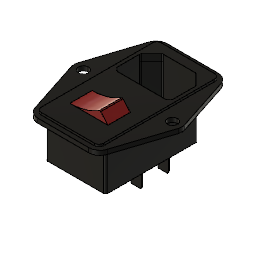
RM PSU Assembly (Autodesk Fusion 360 archive; units mm, degrees)
design "IEC Inlet"
Autodesk Fusion 360 part; units mm, degrees
(part 1 of 2)
sketch "Sketch1" plane through (0, 0, 0) normal (0, 0, 1) x (1, 0, 0)
  line L0 (-25, 14) -> (25, 14)
  line L1 (27, 12) -> (27, -12)
  line L2 (25, -14) -> (-25, -14)
  line L3 (-27, -12) -> (-27, 12)
  arc A0 (-25, 14) -> (-27, 12) centre (-25, 12) ccw
  arc A1 (-27, -12) -> (-25, -14) centre (-25, -12) ccw
  arc A2 (25, -14) -> (27, -12) centre (25, -12) ccw
  arc A3 (27, 12) -> (25, 14) centre (25, 12) ccw
  dimension "d1" = 28
  dimension "d2" = 54
  dimension "d3" = 14
  dimension "d4" = 27
  dimension "d5" = 2
  constraint horizontal L0
  constraint vertical L1
  constraint horizontal L2
  constraint vertical L3
  constraint tangent L3 A0
  constraint tangent L0 A0
  constraint tangent L3 A1
  constraint tangent L2 A1
  constraint equal A0 A1
  constraint tangent L2 A2
  constraint tangent L1 A2
  constraint equal A0 A2
  constraint tangent L1 A3
  constraint tangent L0 A3
  constraint equal A0 A3
  measures "d1" distance of L0 L2
  measures "d2" distance of L1 L3
  measures "d3" distance of origin L2
  measures "d4" distance of origin L3
  measures "d5" radius of A0
extrude "Extrude1" add sketch "Sketch1" along normal blind 1
sketch "Sketch2" plane through (0, 0, 0) normal (0, 0, -1) x (1, 0, 0)
  arc A0 (27, 12) -> (25, 14) centre (25, 12) ccw
  line L0 (25, 14) -> (-25, 14)
  arc A1 (-25, 14) -> (-27, 12) centre (-25, 12) ccw
  line L1 (-27, 12) -> (-27, -12)
  arc A2 (-27, -12) -> (-25, -14) centre (-25, -12) ccw
  line L2 (-25, -14) -> (25, -14)
  arc A3 (25, -14) -> (27, -12) centre (25, -12) ccw
  line L3 (27, -12) -> (27, 12)
  line L4 (-29, 24.5) -> (29, 24.5)
  line L5 (29, 11.423) -> (29, -11.423)
  line L6 (29, -24.5) -> (-29, -24.5)
  line L7 (-29, -11.423) -> (-29, 11.423)
  circle A4 centre (0, -20) radius 2.25
  circle A5 centre (0, 20) radius 2.25
  line L8 (1.5487, -23.9955) -> (25.5487, -16.1771)
  line L9 (-1.5487, -23.9955) -> (-25.5487, -16.1771)
  line L10 (1.5487, 23.9955) -> (25.5487, 16.1771)
  line L11 (-1.5487, 23.9955) -> (-25.5487, 16.1771)
  arc A6 (25.5487, -16.1771) -> (29, -11.423) centre (24, -11.423) ccw
  arc A7 (29, 11.423) -> (25.5487, 16.1771) centre (24, 11.423) ccw
  arc A8 (-25.5487, 16.1771) -> (-29, 11.423) centre (-24, 11.423) ccw
  arc A9 (-29, -11.423) -> (-25.5487, -16.1771) centre (-24, -11.423) ccw
  arc A10 (-1.5487, -23.9955) -> (1.5487, -23.9955) centre (0, -19.2414) ccw
  arc A11 (1.5487, 23.9955) -> (-1.5487, 23.9955) centre (0, 19.2414) ccw
  point P0 (0, -24.5)
  point P1 (29, -15.0528)
  point P2 (-29, -15.0528)
  point P3 (0, 24.5)
  point P4 (29, 15.0528)
  point P5 (-29, 15.0528)
  dimension "d8" = 58
  dimension "d9" = 29
  dimension "d10" = 49
  dimension "d11" = 24.5
  dimension "d12" = 4.5
  dimension "d13" = 4.5
  dimension "d14" = 40
  dimension "d15" = 4.5
  dimension "d16" = 30.5
  dimension "d17" = 30.5
  dimension "d18" = 30.5
  dimension "d19" = 30.5
  dimension "d20" = 5
  dimension "d21" = 5
  constraint horizontal L4
  constraint vertical L5
  constraint horizontal L6
  constraint vertical L7
  constraint vertical origin A5.centre
  constraint vertical origin A4.centre
  constraint midpoint L6 P0
  constraint coincident L5 P1
  constraint coincident L7 P2
  constraint midpoint L4 P3
  constraint coincident L5 P4
  constraint coincident L7 P5
  constraint coincident P1 L8
  constraint coincident L6.start L5
  constraint tangent L8 A6
  constraint tangent L5 A6
  constraint coincident L4.end L5
  constraint coincident P4 L10
  constraint tangent L5 A7
  constraint tangent L10 A7
  constraint equal A6 A7
  constraint coincident P5 L11
  constraint coincident L4.start L7
  constraint tangent L11 A8
  constraint tangent L7 A8
  constraint equal A6 A8
  constraint coincident L6.end L7
  constraint coincident P2 L9
  constraint tangent L7 A9
  constraint tangent L9 A9
  constraint equal A6 A9
  constraint coincident P0 L9
  constraint coincident P0 L8
  constraint tangent L9 A10
  constraint tangent L8 A10
  constraint coincident P3 L10
  constraint coincident P3 L11
  constraint tangent L10 A11
  constraint tangent L11 A11
  constraint equal A10 A11
  measures "d8" distance of L5 L7
  measures "d9" distance of origin L7
  measures "d10" distance of L4 L6
  measures "d11" distance of origin L6
  measures "d12" diameter of A4
  measures "d13" diameter of A5
  measures "d14" distance of A4.centre A5.centre
  measures "d15" distance of L6 A4.centre
  measures "d16" distance of P0 P1
  measures "d17" distance of P0 P2
  measures "d18" distance of P3 P4
  measures "d19" distance of P3 P5
  measures "d20" radius of A6
  measures "d21" radius of A10
extrude "Extrude2" add sketch "Sketch2" along normal blind 2 contours A0 L0 A1 L1 A2 L2 A3 L3 | L5 L7 L8 L9 L10 L11 A6 A7 A8 A9 A10 A11
sketch "Sketch3" plane through (0, 0, -2) normal (0, 0, -1) x (1, 0, 0)
  circle A0 centre (0, 20) radius 2.25
  circle A1 centre (0, -20) radius 2.25
  arc A2 (29, 11.423) -> (25.5487, 16.1771) centre (24, 11.423) ccw
  line L0 (25.5487, 16.1771) -> (1.5487, 23.9955)
  arc A3 (1.5487, 23.9955) -> (-1.5487, 23.9955) centre (0, 19.2414) ccw
  line L1 (-1.5487, 23.9955) -> (-25.5487, 16.1771)
  arc A4 (-25.5487, 16.1771) -> (-29, 11.423) centre (-24, 11.423) ccw
  line L2 (-29, 11.423) -> (-29, -11.423)
  arc A5 (-29, -11.423) -> (-25.5487, -16.1771) centre (-24, -11.423) ccw
  line L3 (-25.5487, -16.1771) -> (-1.5487, -23.9955)
  arc A6 (-1.5487, -23.9955) -> (1.5487, -23.9955) centre (0, -19.2414) ccw
  line L4 (1.5487, -23.9955) -> (25.5487, -16.1771)
  arc A7 (25.5487, -16.1771) -> (29, -11.423) centre (24, -11.423) ccw
  line L5 (29, -11.423) -> (29, 11.423)
  line L6 (-22.5, 13.5) -> (22.5, 13.5)
  line L7 (23.5, 12.5) -> (23.5, -12.5)
  line L8 (22.5, -13.5) -> (-22.5, -13.5)
  line L9 (-23.5, -12.5) -> (-23.5, 12.5)
  arc A8 (23.5, 12.5) -> (22.5, 13.5) centre (22.5, 12.5) ccw
  arc A9 (22.5, -13.5) -> (23.5, -12.5) centre (22.5, -12.5) ccw
  arc A10 (-23.5, -12.5) -> (-22.5, -13.5) centre (-22.5, -12.5) ccw
  arc A11 (-22.5, 13.5) -> (-23.5, 12.5) centre (-22.5, 12.5) ccw
  dimension "d24" = 27
  dimension "d25" = 47
  dimension "d26" = 23.5
  dimension "d27" = 13.5
  dimension "d30" = 1
  constraint horizontal L6
  constraint vertical L7
  constraint horizontal L8
  constraint vertical L9
  constraint tangent L6 A8
  constraint tangent L7 A8
  constraint tangent L7 A9
  constraint tangent L8 A9
  constraint equal A8 A9
  constraint tangent L8 A10
  constraint tangent L9 A10
  constraint equal A8 A10
  constraint tangent L9 A11
  constraint tangent L6 A11
  constraint equal A8 A11
  measures "d24" distance of L6 L8
  measures "d25" distance of L7 L9
  measures "d26" distance of origin L9
  measures "d27" distance of origin L6
  measures "d30" radius of A8
extrude "Extrude3" add sketch "Sketch3" along normal blind 18 contours L6 L7 L8 L9 A8 A9 A10 A11
sketch "Sketch4" plane through (0, 0, -20) normal (0, 0, -1) x (1, 0, 0)
  arc A0 (23.5, 12.5) -> (22.5, 13.5) centre (22.5, 12.5) ccw
  line L0 (22.5, 13.5) -> (-22.5, 13.5)
  arc A1 (-22.5, 13.5) -> (-23.5, 12.5) centre (-22.5, 12.5) ccw
  line L1 (-23.5, 12.5) -> (-23.5, -12.5)
  arc A2 (-23.5, -12.5) -> (-22.5, -13.5) centre (-22.5, -12.5) ccw
  line L2 (-22.5, -13.5) -> (22.5, -13.5)
  arc A3 (22.5, -13.5) -> (23.5, -12.5) centre (22.5, -12.5) ccw
  line L3 (23.5, -12.5) -> (23.5, 12.5)
  line L4 (17.136, 13.5) -> (23.5, 7.136)
  line L5 (23.5, -7.136) -> (17.136, -13.5)
  dimension "d31" = 9
  dimension "d32" = 9
  dimension "d33" = 45
  dimension "d34" = 45
  constraint coincident L0 L4.start
  constraint coincident L3 L4.end
  constraint coincident L3 L5.start
  constraint coincident L2 L5.end
  measures "d31" distance of L5.start L5.end
  measures "d32" distance of L4.start L4.end
  measures "d33" angle of L3 L4
  measures "d34" angle of L3 L5
extrude "Extrude4" cut sketch "Sketch4" against normal blind 18 contours A0 L0 L3 L4 | L2 A3 L3 L5
sketch "Sketch5" plane through (0, 0, 1) normal (0, 0, 1) x (-1, 0, 0)
  arc A0 (-25, 14) -> (-27, 12) centre (-25, 12) ccw
  line L0 (-27, 12) -> (-27, -12)
  arc A1 (-27, -12) -> (-25, -14) centre (-25, -12) ccw
  line L1 (-25, -14) -> (25, -14)
  arc A2 (25, -14) -> (27, -12) centre (25, -12) ccw
  line L2 (27, -12) -> (27, 12)
  arc A3 (27, 12) -> (25, 14) centre (25, 12) ccw
  line L3 (25, 14) -> (-25, 14)
  line L4 (-8, -12.5) -> (-17.636, -12.5)
  line L5 (-23, -7.136) -> (-23, 7.136)
  line L6 (-17.636, 12.5) -> (-8, 12.5)
  line L7 (-6, 10.5) -> (-6, -10.5)
  line L8 (-18.3431, 12.2071) -> (-22.7071, 7.8431)
  line L9 (-22.7071, -7.8431) -> (-18.3431, -12.2071)
  arc A4 (-8, -12.5) -> (-6, -10.5) centre (-8, -10.5) ccw
  arc A5 (-6, 10.5) -> (-8, 12.5) centre (-8, 10.5) ccw
  arc A6 (-18.3431, -12.2071) -> (-17.636, -12.5) centre (-17.636, -11.5) ccw
  arc A7 (-23, -7.136) -> (-22.7071, -7.8431) centre (-22, -7.136) ccw
  arc A8 (-22.7071, 7.8431) -> (-23, 7.136) centre (-22, 7.136) ccw
  arc A9 (-17.636, 12.5) -> (-18.3431, 12.2071) centre (-17.636, 11.5) ccw
  point P0 (-18.0503, 12.5)
  point P1 (-23, 7.5503)
  point P2 (-23, -7.5503)
  point P3 (-18.0503, -12.5)
  dimension "d37" = 4
  dimension "d38" = 17
  dimension "d39" = 25
  dimension "d40" = 12.5
  dimension "d41" = 7
  dimension "d42" = 7
  dimension "d43" = 45
  dimension "d44" = 45
  dimension "d45" = 2
  dimension "d46" = 1
  constraint horizontal L4
  constraint vertical L5
  constraint horizontal L6
  constraint vertical L7
  constraint coincident L6 P0
  constraint coincident L5 P1
  constraint coincident L5 P2
  constraint coincident L4 P3
  constraint tangent L4 A4
  constraint tangent L7 A4
  constraint tangent L6 A5
  constraint tangent L7 A5
  constraint equal A4 A5
  constraint coincident P3 L9
  constraint tangent L4 A6
  constraint tangent L9 A6
  constraint coincident P2 L9
  constraint tangent L9 A7
  constraint tangent L5 A7
  constraint equal A6 A7
  constraint coincident P1 L8
  constraint tangent L5 A8
  constraint tangent L8 A8
  constraint equal A6 A8
  constraint coincident P0 L8
  constraint tangent L8 A9
  constraint tangent L6 A9
  constraint equal A6 A9
  measures "d37" distance of L0 L5
  measures "d38" distance of L5 L7
  measures "d39" distance of L4 L6
  measures "d40" distance of origin L6
  measures "d41" distance of P0 P1
  measures "d42" distance of P2 P3
  measures "d43" angle of L5 L9
  measures "d44" angle of L5 L8
  measures "d45" radius of A4
  measures "d46" radius of A6
extrude "Extrude5" cut sketch "Sketch5" against normal blind 18 contours L4 L5 L6 L7 L8 L9 A4 A5 A6 A7 A8 A9
sketch "Sketch6" plane through (0, 0, 1) normal (0, 0, 1) x (-1, 0, 0)
  line L0 (-17.636, 12.5) -> (-8, 12.5)
  arc A0 (-6, 10.5) -> (-8, 12.5) centre (-8, 10.5) ccw
  line L1 (-6, 10.5) -> (-6, -10.5)
  arc A1 (-8, -12.5) -> (-6, -10.5) centre (-8, -10.5) ccw
  line L2 (-8, -12.5) -> (-17.636, -12.5)
  arc A2 (-18.3431, -12.2071) -> (-17.636, -12.5) centre (-17.636, -11.5) ccw
  line L3 (-18.3431, -12.2071) -> (-22.7071, -7.8431)
  arc A3 (-23, -7.136) -> (-22.7071, -7.8431) centre (-22, -7.136) ccw
  line L4 (-23, -7.136) -> (-23, 7.136)
  arc A4 (-22.7071, 7.8431) -> (-23, 7.136) centre (-22, 7.136) ccw
  line L5 (-22.7071, 7.8431) -> (-18.3431, 12.2071)
  arc A5 (-17.636, 12.5) -> (-18.3431, 12.2071) centre (-17.636, 11.5) ccw
  arc A6 (-25, 14) -> (-27, 12) centre (-25, 12) ccw
  line L6 (-27, 12) -> (-27, -12)
  arc A7 (-27, -12) -> (-25, -14) centre (-25, -12) ccw
  line L7 (-25, -14) -> (25, -14)
  arc A8 (25, -14) -> (27, -12) centre (25, -12) ccw
  line L8 (27, -12) -> (27, 12)
  arc A9 (27, 12) -> (25, 14) centre (25, 12) ccw
  line L9 (25, 14) -> (-25, 14)
  line L10 (17, -8) -> (7, -8)
  line L11 (7, -8) -> (7, 8)
  line L12 (7, 8) -> (17, 8)
  line L13 (17, 8) -> (17, -8)
  line L14 (17, 4.5) -> (7, 4.5)
  dimension "d49" = 16
  dimension "d50" = 10
  dimension "d51" = 10
  dimension "d52" = 6
  dimension "d53" = 12.5
  constraint horizontal L10
  constraint vertical L11
  constraint horizontal L12
  constraint vertical L13
  constraint coincident L13 L14.start
  constraint coincident L11 L14.end
  constraint perpendicular L11 L14
  measures "d49" distance of L10 L12
  measures "d50" distance of L11 L13
  measures "d51" distance of L8 L13
  measures "d52" distance of L7 L10
  measures "d53" distance of L10 L14
extrude "Extrude6" add sketch "Sketch6" along normal blind 4 contours L11 L12 L13 L14
fillet "Fillet1" radius 25 1 edges at (-12, -4.5, 1)
sketch "Sketch7" plane through (-17, 0, 0) normal (-1, 0, 0) x (0, -1, 0)
  line L0 (-9.0647, 1) -> (8, 1)
  line L1 (8, 1) -> (8, 5)
  line L2 (8, 5) -> (4.5, 5)
  arc A0 (-9.0647, 1) -> (4.5, 5) centre (-9.0647, 26) ccw
  line L3 (4.5, 5) -> (8, 1)
  constraint coincident L2.end A0.end
  constraint coincident L0.end L1.start
extrude "Extrude7" cut sketch "Sketch7" against normal blind 10 contours L1 L2 L3
fillet "Fillet2" radius 0.5 1 edges at (-12, -4.5, 5)
sketch "Sketch9" plane through (0, 0, -20) normal (0, 0, -1) x (1, 0, 0)
  line L0 (23.5, 7.136) -> (17.136, 13.5)
  line L1 (17.136, 13.5) -> (-22.5, 13.5)
  arc A0 (-22.5, 13.5) -> (-23.5, 12.5) centre (-22.5, 12.5) ccw
  line L2 (-23.5, 12.5) -> (-23.5, -12.5)
  arc A1 (-23.5, -12.5) -> (-22.5, -13.5) centre (-22.5, -12.5) ccw
  line L3 (-22.5, -13.5) -> (17.136, -13.5)
  line L4 (17.136, -13.5) -> (23.5, -7.136)
  line L5 (23.5, -7.136) -> (23.5, 7.136)
  line L6 (-21.5, 12.5) -> (-8.5, 12.5)
  line L7 (-7.5, 11.5) -> (-7.5, -11.5)
  line L8 (-8.5, -12.5) -> (-21.5, -12.5)
  line L9 (-22.5, -11.5) -> (-22.5, 11.5)
  arc A2 (-21.5, 12.5) -> (-22.5, 11.5) centre (-21.5, 11.5) ccw
  arc A3 (-7.5, 11.5) -> (-8.5, 12.5) centre (-8.5, 11.5) ccw
  arc A4 (-8.5, -12.5) -> (-7.5, -11.5) centre (-8.5, -11.5) ccw
  arc A5 (-22.5, -11.5) -> (-21.5, -12.5) centre (-21.5, -11.5) ccw
  dimension "d62" = 1
  dimension "d63" = 1
  dimension "d64" = 1
  dimension "d65" = 15
  dimension "d66" = 1
  constraint horizontal L6
  constraint vertical L7
  constraint horizontal L8
  constraint vertical L9
  constraint tangent L6 A2
  constraint tangent L9 A2
  constraint tangent L6 A3
  constraint tangent L7 A3
  constraint equal A2 A3
  constraint tangent L7 A4
  constraint tangent L8 A4
  constraint equal A2 A4
  constraint tangent L8 A5
  constraint tangent L9 A5
  constraint equal A2 A5
  measures "d62" distance of L1 L6
  measures "d63" distance of L3 L8
  measures "d64" distance of L2 L9
  measures "d65" distance of L7 L9
  measures "d66" radius of A2
extrude "Extrude8" cut sketch "Sketch9" against normal blind 18 contours L6 L7 L8 L9 A2 A3 A4 A5
sketch "Sketch10" plane through (0, 0, -20) normal (0, 0, -1) x (1, 0, 0)
  line L0 (-22.5, -11.5) -> (-22.5, 11.5)
  arc A0 (-21.5, 12.5) -> (-22.5, 11.5) centre (-21.5, 11.5) ccw
  line L1 (-21.5, 12.5) -> (-8.5, 12.5)
  arc A1 (-7.5, 11.5) -> (-8.5, 12.5) centre (-8.5, 11.5) ccw
  line L2 (-7.5, 11.5) -> (-7.5, -11.5)
  arc A2 (-8.5, -12.5) -> (-7.5, -11.5) centre (-8.5, -11.5) ccw
  line L3 (-8.5, -12.5) -> (-21.5, -12.5)
  arc A3 (-22.5, -11.5) -> (-21.5, -12.5) centre (-21.5, -11.5) ccw
  line L4 (23.5, 7.136) -> (17.136, 13.5)
  line L5 (17.136, 13.5) -> (-22.5, 13.5)
  arc A4 (-22.5, 13.5) -> (-23.5, 12.5) centre (-22.5, 12.5) ccw
  line L6 (-23.5, 12.5) -> (-23.5, -12.5)
  arc A5 (-23.5, -12.5) -> (-22.5, -13.5) centre (-22.5, -12.5) ccw
  line L7 (-22.5, -13.5) -> (17.136, -13.5)
  line L8 (17.136, -13.5) -> (23.5, -7.136)
  line L9 (23.5, -7.136) -> (23.5, 7.136)
  line L10 (19.5, 2.5) -> (20, 2.5)
  line L11 (20, 2.5) -> (20, -2.5)
  line L12 (20, -2.5) -> (19.5, -2.5)
  line L13 (19.5, -2.5) -> (19.5, 2.5)
  line L14 (8.636, 9.5) -> (9.136, 9.5)
  line L15 (9.136, 9.5) -> (9.136, 4.5)
  line L16 (9.136, 4.5) -> (8.636, 4.5)
  line L17 (8.636, 4.5) -> (8.636, 9.5)
  line L18 (-3.364, 9.5) -> (-2.864, 9.5)
  line L19 (-2.864, 9.5) -> (-2.864, 4.5)
  line L20 (-2.864, 4.5) -> (-3.364, 4.5)
  line L21 (-3.364, 4.5) -> (-3.364, 9.5)
  dimension "d69" = 5
  dimension "d70" = 0.5
  dimension "d71" = 0.5
  dimension "d72" = 5
  dimension "d75" = 3.5
  dimension "d76" = 11
  dimension "d77" = 4
  dimension "d78" = 5
  dimension "d79" = 0.5
  dimension "d80" = 4
  dimension "d81" = 8
  dimension "d82" = 20
  constraint horizontal L10
  constraint vertical L11
  constraint horizontal L12
  constraint vertical L13
  constraint horizontal L14
  constraint vertical L15
  constraint horizontal L16
  constraint vertical L17
  constraint horizontal L18
  constraint vertical L19
  constraint horizontal L20
  constraint vertical L21
  measures "d69" distance of L10 L12
  measures "d70" distance of L11 L13
  measures "d71" distance of L15 L17
  measures "d72" distance of L14 L16
  measures "d75" distance of L9 L11
  measures "d76" distance of L7 L12
  measures "d77" distance of L5 L14
  measures "d78" distance of L18 L20
  measures "d79" distance of L19 L21
  measures "d80" distance of L5 L18
  measures "d81" distance of L4.end L15
  measures "d82" distance of L4.end L19
extrude "Extrude9" add sketch "Sketch10" along normal blind 10 contours L10 L11 L12 L13 | L14 L15 L16 L17 | L18 L19 L20 L21
sketch "Sketch11" plane through (-3.364, 0, 0) normal (-1, 0, 0) x (0, -1, 0)
  line L0 (9.5, -20) -> (4.5, -20)
  line L1 (4.5, -20) -> (4.5, -30)
  line L2 (4.5, -30) -> (9.5, -30)
  line L3 (9.5, -30) -> (9.5, -20)
  line L4 (5, -30) -> (4.5, -29.134)
  line L5 (9, -30) -> (9.5, -29.134)
  dimension "d85" = 1
  dimension "d86" = 1
  dimension "d87" = 30
  dimension "d88" = 30
  constraint coincident L2 L4.start
  constraint coincident L1 L4.end
  constraint coincident L2 L5.start
  constraint coincident L3 L5.end
  measures "d85" distance of L5.start L5.end
  measures "d86" distance of L4.start L4.end
  measures "d87" angle of L3 L5
  measures "d88" angle of L1 L4
extrude "Extrude10" cut sketch "Sketch11" against normal blind 15 contours L2 L3 L5 | L1 L2 L4
sketch "Sketch12" plane through (19.5, 0, 0) normal (-1, 0, 0) x (0, -1, 0)
  line L0 (2.5, -20) -> (-2.5, -20)
  line L1 (-2.5, -20) -> (-2.5, -30)
  line L2 (-2.5, -30) -> (2.5, -30)
  line L3 (2.5, -30) -> (2.5, -20)
  line L4 (2.5, -29.134) -> (2, -30)
  line L5 (-2, -30) -> (-2.5, -29.134)
  dimension "d91" = 1
  dimension "d92" = 1
  dimension "d93" = 30
  dimension "d94" = 30
  constraint coincident L3 L4.start
  constraint coincident L2 L4.end
  constraint coincident L2 L5.start
  constraint coincident L1 L5.end
  measures "d91" distance of L5.start L5.end
  measures "d92" distance of L4.start L4.end
  measures "d93" angle of L3 L4
  measures "d94" angle of L1 L5
extrude "Extrude11" cut sketch "Sketch12" against normal blind 0.5 contours L2 L3 L4 | L1 L2 L5
sketch "Sketch13" plane through (0, 0, -20) normal (0, 0, -1) x (1, 0, 0)
  line L0 (19.5, -2.5) -> (19.5, 2.5)
  line L1 (19.5, 2.5) -> (20, 2.5)
  line L2 (20, 2.5) -> (20, -2.5)
  line L3 (20, -2.5) -> (19.5, -2.5)
  line L4 (8.636, 4.5) -> (8.636, 9.5)
  line L5 (8.636, 9.5) -> (9.136, 9.5)
  line L6 (9.136, 9.5) -> (9.136, 4.5)
  line L7 (9.136, 4.5) -> (8.636, 4.5)
  line L8 (-3.364, 4.5) -> (-3.364, 9.5)
  line L9 (-3.364, 9.5) -> (-2.864, 9.5)
  line L10 (-2.864, 9.5) -> (-2.864, 4.5)
  line L11 (-2.864, 4.5) -> (-3.364, 4.5)
  line L12 (-22.5, -11.5) -> (-22.5, 11.5)
  arc A0 (-21.5, 12.5) -> (-22.5, 11.5) centre (-21.5, 11.5) ccw
  line L13 (-21.5, 12.5) -> (-8.5, 12.5)
  arc A1 (-7.5, 11.5) -> (-8.5, 12.5) centre (-8.5, 11.5) ccw
  line L14 (-7.5, 11.5) -> (-7.5, -11.5)
  arc A2 (-8.5, -12.5) -> (-7.5, -11.5) centre (-8.5, -11.5) ccw
  line L15 (-8.5, -12.5) -> (-21.5, -12.5)
  arc A3 (-22.5, -11.5) -> (-21.5, -12.5) centre (-21.5, -11.5) ccw
  line L16 (23.5, 7.136) -> (17.136, 13.5)
  line L17 (17.136, 13.5) -> (-22.5, 13.5)
  arc A4 (-22.5, 13.5) -> (-23.5, 12.5) centre (-22.5, 12.5) ccw
  line L18 (-23.5, 12.5) -> (-23.5, -12.5)
  arc A5 (-23.5, -12.5) -> (-22.5, -13.5) centre (-22.5, -12.5) ccw
  line L19 (-22.5, -13.5) -> (17.136, -13.5)
  line L20 (17.136, -13.5) -> (23.5, -7.136)
  line L21 (23.5, -7.136) -> (23.5, 7.136)
  line L22 (17.0773, 5.378) -> (22.5771, 5.378)
  line L23 (22.5771, 5.378) -> (22.5771, -4.9703)
  line L24 (22.5771, -4.9703) -> (17.0773, -4.9703)
  line L25 (17.0773, -4.9703) -> (17.0773, 5.378)
  constraint horizontal L22
  constraint vertical L23
  constraint horizontal L24
  constraint vertical L25
extrude "Extrude12" [suppressed]
equation "d3 = ( 28 / 2 ) * 1 mm"
equation "d4 = ( 54 / 2 ) * 1 mm"
equation "d9 = ( 58 / 2 ) * 1 mm"
equation "d11 = ( 49 / 2 ) * 1 mm"
equation "d26 = ( 47 / 2 ) * 1 mm"
equation "d27 = ( 27 / 2 ) * 1 mm"
equation "d40 = ( 25 / 2 ) * 1 mm"
equation "d76 = ( 27 / 2 ) * 1 mm - 2.5 mm"

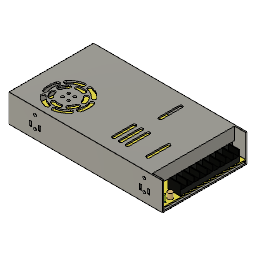
design "LRS-600-36"
Autodesk Fusion 360 part; units mm, degrees
sketch "Sketch1" plane through (0, 0, 0) normal (0, 0, 1) x (1, 0, 0)
  line L0 (62, 112.5) -> (-62, 112.5)
  line L1 (-62, 112.5) -> (-62, -112.5)
  line L2 (-62, -112.5) -> (62, -112.5)
  line L3 (62, -112.5) -> (62, 112.5)
  line L4 (62, 112.5) -> (-62, -112.5) construction
  line L5 (-62, 112.5) -> (62, -112.5) construction
  dimension "d1" = 124
  dimension "d2" = 225
  constraint horizontal L0
  constraint perpendicular L0 L1
  constraint parallel L0 L2
  constraint parallel L1 L3
  constraint coincident L4 origin
  constraint coincident L5 origin
  measures "d1" distance of L1.end L2.end
  measures "d2" distance of L0.end L1.end
extrude "Extrude1" add sketch "Sketch1" along normal blind 41 makes body 1
sketch "Sketch2" plane through (62, 0, 0) normal (1, 0, 0) x (0, 1, 0)
  line L0 (-112.5, 0) -> (112.5, 0)
  line L1 (112.5, 0) -> (112.5, 41)
  line L2 (112.5, 41) -> (-112.5, 41)
  line L3 (-112.5, 41) -> (-112.5, 0)
  circle A0 centre (-85.8, 31) radius 2
  circle A1 centre (-85.8, 13) radius 2
  circle A2 centre (74.2, 31) radius 2
  circle A3 centre (74.2, 13) radius 2
  line L4 (-85.8, 0) -> (-85.8, 41) construction
  line L5 (74.2, 0) -> (74.2, 41) construction
  line L6 (-85.8, 31) -> (74.2, 31) construction
  line L7 (-85.8, 13) -> (74.2, 13) construction
  dimension "d5" = 4
  dimension "d6" = 26.7
  dimension "d7" = 160
  dimension "d8" = 13
  dimension "d9" = 18
  constraint equal A0 A1
  constraint equal A1 A2
  constraint equal A2 A3
  constraint coincident L0 L4.start
  constraint coincident L2 L4.end
  constraint perpendicular L2 L4
  constraint coincident L0 L5.start
  constraint coincident L2 L5.end
  constraint perpendicular L2 L5
  constraint coincident A0.centre L4
  constraint coincident A1.centre L4
  constraint coincident A2.centre L5
  constraint coincident A3.centre L5
  constraint coincident A0.centre L6.start
  constraint coincident L5 A2.centre
  constraint perpendicular L5 L6
  constraint coincident A1.centre L7.start
  constraint coincident L5 A3.centre
  constraint perpendicular L5 L7
  constraint coincident A2.centre L6
  constraint coincident A3.centre L7
  measures "d5" diameter of A0
  measures "d6" distance of L3 L4
  measures "d7" distance of L4 L5
  measures "d8" distance of A1.centre L4.start
  measures "d9" distance of A0.centre A1.centre
shell "Shell1" thickness 2 removed faces 0 bodies 1
extrude "Extrude2" cut sketch "Sketch2" against normal through all contours A0 | A1 | A2 | A3 bodies 1
sketch "Sketch3" plane through (0, 0, 41) normal (0, 0, 1) x (-1, 0, 0)
  line L0 (-62, 112.5) -> (-62, -112.5)
  line L1 (-62, -112.5) -> (62, -112.5)
  line L2 (62, -112.5) -> (62, 112.5)
  line L3 (62, 112.5) -> (-62, 112.5)
  line L4 (62, 96.1) -> (-62, 96.1)
  line L5 (-60, 112.5) -> (-60, 96.1)
  line L6 (60, 96.1) -> (60, 112.5)
  dimension "d12" = 16.4
  constraint coincident L2 L4.start
  constraint coincident L0 L4.end
  constraint perpendicular L0 L4
  constraint coincident L4 L6.start
  constraint coincident L4 L5.end
  measures "d12" distance of L3 L4
extrude "Extrude3" cut sketch "Sketch3" against normal up to surface (39 mm away) contours L3 L4 L5 L6 bodies 1
sketch "Sketch4" plane through (0, 0, 0) normal (0, 0, -1) x (1, 0, 0)
  line L0 (62, -112.5) -> (62, 112.5)
  line L1 (62, 112.5) -> (-62, 112.5)
  line L2 (-62, 112.5) -> (-62, -112.5)
  line L3 (-62, -112.5) -> (62, -112.5)
  line L4 (25.5, 79) -> (-24.5, 79) construction
  line L5 (-24.5, 79) -> (-24.5, -71) construction
  line L6 (-24.5, -71) -> (25.5, -71) construction
  line L7 (25.5, -71) -> (25.5, 79) construction
  circle A0 centre (-24.5, 79) radius 2
  circle A1 centre (25.5, 79) radius 2
  circle A2 centre (25.5, -71) radius 2
  circle A3 centre (-24.5, -71) radius 2
  dimension "d18" = 150
  dimension "d19" = 50
  dimension "d21" = 33.5
  dimension "d22" = 37.5
  dimension "d23" = 4
  constraint horizontal L4
  constraint vertical L5
  constraint horizontal L6
  constraint vertical L7
  constraint coincident L4.end L5.start
  constraint coincident L4.start L7.end
  constraint coincident L6.end L7.start
  constraint coincident L5.end L6.start
  constraint equal A0 A1
  constraint equal A1 A2
  constraint equal A2 A3
  measures "d18" distance of L4.start L6.end
  measures "d19" distance of L4.start L4.end
  measures "d21" distance of L1 L4
  measures "d22" distance of L2 L5
  measures "d23" diameter of A0
extrude "Extrude4" cut sketch "Sketch4" against normal blind 2 contours A0 | A1 | A2 | A3 bodies 1
sketch "Sketch5" plane through (0, 0, 2) normal (0, 0, 1) x (-1, 0, 0)
  circle A0 centre (24.5, 79) radius 2
  circle A1 centre (-25.5, -71) radius 2
  circle A2 centre (-25.5, 79) radius 2
  circle A3 centre (24.5, -71) radius 2
  line L0 (-60, 112.5) -> (-60, -110.5)
  line L1 (-60, -110.5) -> (60, -110.5)
  line L2 (60, -110.5) -> (60, 112.5)
  line L3 (60, 112.5) -> (-60, 112.5)
extrude "Extrude5" add sketch "Sketch5" along normal blind 1.7 from surface at 3 separate body contours A0 | A1 | A2 | A3 | L0 L1 L2 L3 makes body 2
sketch "Sketch6" plane through (0, 0, 6.7) normal (0, 0, 1) x (-1, 0, 0)
  line L0 (60, 112.5) -> (-60, 112.5)
  line L1 (-60, 112.5) -> (-60, -110.5)
  line L2 (-60, -110.5) -> (60, -110.5)
  line L3 (60, -110.5) -> (60, 112.5)
  line L4 (-52.7, 110.9) -> (34.3, 110.9)
  line L5 (34.3, 110.9) -> (34.3, 92.9)
  line L6 (34.3, 92.9) -> (-52.7, 92.9)
  line L7 (-52.7, 92.9) -> (-52.7, 110.9)
  dimension "d29" = 87
  dimension "d30" = 18
  dimension "d31" = 1.6
  dimension "d32" = 7.3
  constraint horizontal L4
  constraint vertical L5
  constraint horizontal L6
  constraint vertical L7
  measures "d29" distance of L4.start L4.end
  measures "d30" distance of L4.start L6.end
  measures "d31" distance of L0 L4
  measures "d32" distance of L1 L7
extrude "Extrude6" add sketch "Sketch6" along normal blind 15.4 separate body contours L4 L5 L6 L7 makes body 3
sketch "Sketch7" plane through (0, 0, 6.7) normal (0, 0, 1) x (-1, 0, 0)
  line L0 (60, 112.5) -> (-60, 112.5)
  line L1 (-60, 112.5) -> (-60, -110.5)
  line L2 (-60, -110.5) -> (60, -110.5)
  line L3 (60, -110.5) -> (60, 112.5)
  circle A0 centre (44, 106) radius 3.5
  circle A1 centre (53.5, 107) radius 1.5
  dimension "d35" = 3
  dimension "d36" = 7
  dimension "d37" = 6.5
  dimension "d38" = 5.5
  dimension "d39" = 6.5
  dimension "d40" = 16
  measures "d35" diameter of A1
  measures "d36" diameter of A0
  measures "d37" distance of L3 A1.centre
  measures "d38" distance of L0 A1.centre
  measures "d39" distance of L0 A0.centre
  measures "d40" distance of L3 A0.centre
extrude "Extrude7" add sketch "Sketch7" along normal blind 10 contours A1 bodies 2
extrude "Extrude8" add sketch "Sketch7" along normal blind 8 contours A0 bodies 2
sketch "Sketch8" plane through (0, 0, 22.1) normal (0, 0, 1) x (-1, 0, 0)
  line L0 (-52.7, 92.9) -> (34.3, 92.9)
  line L1 (34.3, 92.9) -> (34.3, 110.9)
  line L2 (34.3, 110.9) -> (-52.7, 110.9)
  line L3 (-52.7, 110.9) -> (-52.7, 92.9)
  line L4 (-52.7, 110.9) -> (-51.5, 110.9)
  line L5 (-51.5, 110.9) -> (-51.5, 95.9)
  line L6 (-51.5, 95.9) -> (-43.3, 95.9)
  line L7 (-43.3, 95.9) -> (-43.3, 110.9)
  line L8 (-41.95, 110.9) -> (-41.95, 95.9)
  line L9 (-41.95, 95.9) -> (-33.75, 95.9)
  line L10 (-33.75, 95.9) -> (-33.75, 110.9)
  line L11 (-32.4, 110.9) -> (-32.4, 95.9)
  line L12 (-32.4, 95.9) -> (-24.2, 95.9)
  line L13 (-24.2, 95.9) -> (-24.2, 110.9)
  line L14 (-22.85, 110.9) -> (-22.85, 95.9)
  line L15 (-22.85, 95.9) -> (-14.65, 95.9)
  line L16 (-14.65, 95.9) -> (-14.65, 110.9)
  line L17 (-13.3, 110.9) -> (-13.3, 95.9)
  line L18 (-13.3, 95.9) -> (-5.1, 95.9)
  line L19 (-5.1, 95.9) -> (-5.1, 110.9)
  line L20 (-3.75, 110.9) -> (-3.75, 95.9)
  line L21 (-3.75, 95.9) -> (4.45, 95.9)
  line L22 (4.45, 95.9) -> (4.45, 110.9)
  line L23 (5.8, 110.9) -> (5.8, 95.9)
  line L24 (5.8, 95.9) -> (14, 95.9)
  line L25 (14, 95.9) -> (14, 110.9)
  line L26 (15.35, 110.9) -> (15.35, 95.9)
  line L27 (15.35, 95.9) -> (23.55, 95.9)
  line L28 (23.55, 95.9) -> (23.55, 110.9)
  line L29 (24.9, 110.9) -> (24.9, 95.9)
  line L30 (24.9, 95.9) -> (33.1, 95.9)
  line L31 (33.1, 95.9) -> (33.1, 110.9)
  line L32 (24.9, 110.9) -> (23.55, 110.9)
  line L33 (15.35, 110.9) -> (14, 110.9)
  line L34 (5.8, 110.9) -> (4.45, 110.9)
  line L35 (-3.75, 110.9) -> (-5.1, 110.9)
  line L36 (-13.3, 110.9) -> (-14.65, 110.9)
  line L37 (-22.85, 110.9) -> (-24.2, 110.9)
  line L38 (-32.4, 110.9) -> (-33.75, 110.9)
  line L39 (-41.95, 110.9) -> (-43.3, 110.9)
  line L40 (34.3, 110.9) -> (33.1, 110.9)
  dimension "d45" = 8.2
  dimension "d46" = 1.35
  dimension "d47" = 15
  constraint coincident L2.end L3.start
  constraint coincident L2 L4.end
  constraint perpendicular L3 L4
  constraint perpendicular L4 L5
  constraint perpendicular L3 L6
  constraint coincident L2 L7.end
  constraint perpendicular L4 L7
  constraint perpendicular L4 L8
  constraint perpendicular L7 L9
  constraint coincident L2 L10.end
  constraint perpendicular L2 L10
  constraint coincident L2 L11.start
  constraint perpendicular L2 L11
  constraint perpendicular L11 L12
  constraint coincident L2 L13.end
  constraint perpendicular L2 L13
  constraint coincident L2 L14.start
  constraint perpendicular L2 L14
  constraint perpendicular L14 L15
  constraint coincident L2 L16.end
  constraint perpendicular L2 L16
  constraint coincident L2 L17.start
  constraint perpendicular L2 L17
  constraint perpendicular L17 L18
  constraint coincident L2 L19.end
  constraint perpendicular L2 L19
  constraint coincident L2 L20.start
  constraint perpendicular L2 L20
  constraint perpendicular L19 L21
  constraint coincident L2 L22.end
  constraint perpendicular L21 L22
  constraint coincident L2 L23.start
  constraint perpendicular L2 L23
  constraint perpendicular L19 L24
  constraint coincident L2 L25.end
  constraint perpendicular L2 L25
  constraint coincident L2 L26.start
  constraint perpendicular L2 L26
  constraint perpendicular L26 L27
  constraint coincident L2 L28.end
  constraint perpendicular L2 L28
  constraint coincident L2 L29.start
  constraint perpendicular L2 L29
  constraint perpendicular L29 L30
  constraint coincident L2 L31.end
  constraint perpendicular L2 L31
  constraint equal L27 L30
  constraint equal L24 L27
  constraint equal L21 L24
  constraint equal L18 L21
  constraint equal L15 L18
  constraint equal L12 L15
  constraint equal L9 L12
  constraint equal L6 L9
  constraint perpendicular L8 L39
  constraint equal L38 L39
  constraint equal L37 L38
  constraint equal L36 L37
  constraint equal L35 L36
  constraint equal L34 L35
  constraint equal L33 L34
  constraint equal L32 L33
  constraint coincident L1.end L2.start
  constraint equal L4 L40
  constraint collinear L27 L30
  constraint collinear L24 L27
  constraint collinear L21 L24
  constraint collinear L15 L21
  constraint collinear L15 L18
  constraint collinear L12 L18
  constraint collinear L9 L12
  constraint collinear L6 L9
  measures "d45" distance of L29.end L30.end
  measures "d46" distance of L7.end L8.start
  measures "d47" distance of L4.end L5.end
extrude "Extrude9" cut sketch "Sketch8" against normal blind 8 contours L2 L5 L6 L7 | L2 L29 L30 L31 | L2 L8 L9 L10 | L2 L26 L27 L28 | L2 L11 L12 L13 | L2 L23 L24 L25 | L2 L14 L15 L16 | L2 L20 L21 L22 | L2 L17 L18 L19 bodies 3
sketch "Sketch9" plane through (0, 0, 41) normal (0, 0, 1) x (-1, 0, 0)
  line L0 (-60, 96.1) -> (-60, 112.5)
  line L1 (-60, 112.5) -> (-62, 112.5)
  line L2 (-62, 112.5) -> (-62, -112.5)
  line L3 (-62, -112.5) -> (62, -112.5)
  line L4 (62, -112.5) -> (62, 112.5)
  line L5 (62, 112.5) -> (60, 112.5)
  line L6 (60, 112.5) -> (60, 96.1)
  line L7 (60, 96.1) -> (-60, 96.1)
  circle A0 centre (24.5, -62.5) radius 30 construction
  circle A1 centre (24.5, -62.5) radius 26.5 construction
  circle A2 centre (24.5, -62.5) radius 18.5 construction
  circle A3 centre (24.5, -62.5) radius 21.5
  circle A4 centre (24.5, -62.5) radius 15.5
  circle A5 centre (24.5, -62.5) radius 29.5
  circle A6 centre (24.5, -62.5) radius 23.5
  line L8 (24.5, -62.5) -> (62, -62.5) construction
  line L9 (24.5, -62.5) -> (62, -72.5481) construction
  circle A7 centre (42.3696, -67.2882) radius 3
  circle A8 centre (42.3696, -57.7118) radius 3
  circle A9 centre (37.5815, -49.4185) radius 3
  circle A10 centre (29.2882, -44.6304) radius 3
  circle A11 centre (19.7118, -44.6304) radius 3
  circle A12 centre (11.4185, -49.4185) radius 3
  circle A13 centre (6.6304, -57.7118) radius 3
  circle A14 centre (6.6304, -67.2882) radius 3
  circle A15 centre (11.4185, -75.5815) radius 3
  circle A16 centre (19.7118, -80.3696) radius 3
  circle A17 centre (29.2882, -80.3696) radius 3
  circle A18 centre (37.5815, -75.5815) radius 3
  line L10 (24.5, -62.5) -> (25.2686, -62.7059) construction
  line L11 (24.5, -62.5) -> (62, -69.1123) construction
  circle A19 centre (50.5974, -67.1017) radius 3
  circle A20 centre (50.5974, -57.8983) radius 3
  circle A21 centre (47.4497, -49.25) radius 3
  circle A22 centre (41.5339, -42.1998) radius 3
  circle A23 centre (33.5635, -37.5981) radius 3
  circle A24 centre (24.5, -36) radius 3
  circle A25 centre (15.4365, -37.5981) radius 3
  circle A26 centre (7.4661, -42.1998) radius 3
  circle A27 centre (1.5503, -49.25) radius 3
  circle A28 centre (-1.5974, -57.8983) radius 3
  circle A29 centre (-1.5974, -67.1017) radius 3
  circle A30 centre (1.5503, -75.75) radius 3
  circle A31 centre (7.4661, -82.8002) radius 3
  circle A32 centre (15.4365, -87.4019) radius 3
  circle A33 centre (24.5, -89) radius 3
  circle A34 centre (33.5635, -87.4019) radius 3
  circle A35 centre (41.5339, -82.8002) radius 3
  circle A36 centre (47.4497, -75.75) radius 3
  dimension "d50" = 37.5
  dimension "d51" = 50
  dimension "d52" = 60
  dimension "d53" = 53
  dimension "d54" = 37
  dimension "d55" = 3
  dimension "d56" = -3
  dimension "d57" = 3
  dimension "d58" = -3
  dimension "d59" = 15
  dimension "d61" = 360
  dimension "d62" = 10
  dimension "d64" = 360
  constraint concentric A0 A1
  constraint concentric A0 A2
  constraint coincident A0.centre A1.centre
  constraint perpendicular L4 L8
  constraint coincident L4 L9.end
  constraint coincident L4 L8.end
  constraint coincident A2 A7.centre
  constraint coincident L9 A7.centre
  constraint tangent A4 A7
  constraint coincident L9 L10.end
  constraint coincident L4 L11.end
  constraint coincident A1 A19.centre
  constraint coincident L11 A19.centre
  constraint tangent A6 A19
  measures "d50" distance of L4 A0.centre
  measures "d51" distance of L3 A0.centre
  measures "d52" diameter of A0
  measures "d53" diameter of A1
  measures "d54" diameter of A2
  measures "d59" angle of L8 L9
  measures "d62" angle of L8 L11
extrude "Extrude10" cut sketch "Sketch9" against normal blind 2 contours A3 A4 A7 A8 | A8 | A7 | A3 A4 A9 A10 | A9 | A3 A4 A17 A18 | A18 | A10 | A17 | A3 A4 A11 A12 | A11 | A3 A4 A15 A16 | A16 | A12 | A15 | A3 A4 A13 A14 | A13 | A14 | A5 A6 A20 A21 | A20 | A5 A6 A19 A36 | A19 | A5 A6 A21 A22 | A21 | A5 A6 A35 A36 | A36 | A22 | A35 | A5 A6 A23 A24 | A23 | A5 A6 A33 A34 | A34 | A5 A6 A24 A25 | A24 | A5 A6 A32 A33 | A33 | A25 | A32 | A5 A6 A26 A27 | A26 | A5 A6 A30 A31 | A31 | A5 A6 A27 A28 | A27 | A5 A6 A29 A30 | A30 | A28 | A29 bodies 1
sketch "Sketch10" plane through (0, 0, 41) normal (0, 0, 1) x (-1, 0, 0)
  arc A0 (14.4104, -90.2209) -> (34.5896, -90.2209) centre (24.5, -62.5) ccw
  arc A1 (16.4625, -84.5828) -> (14.4104, -90.2209) centre (15.4365, -87.4019) ccw
  arc A2 (16.4625, -84.5828) -> (32.5375, -84.5828) centre (24.5, -62.5) ccw
  arc A3 (34.5896, -90.2209) -> (32.5375, -84.5828) centre (33.5635, -87.4019) ccw
  arc A4 (18.9354, -41.7326) -> (9.2972, -47.2972) centre (24.5, -62.5) ccw
  arc A5 (20.4883, -47.5281) -> (18.9354, -41.7326) centre (19.7118, -44.6304) ccw
  arc A6 (20.4883, -47.5281) -> (13.5398, -51.5398) centre (24.5, -62.5) ccw
  arc A7 (9.2972, -47.2972) -> (13.5398, -51.5398) centre (11.4185, -49.4185) ccw
  arc A8 (45.2674, -68.0646) -> (45.2674, -56.9354) centre (24.5, -62.5) ccw
  arc A9 (39.4719, -66.5117) -> (45.2674, -68.0646) centre (42.3696, -67.2882) ccw
  arc A10 (39.4719, -66.5117) -> (39.4719, -58.4883) centre (24.5, -62.5) ccw
  arc A11 (45.2674, -56.9354) -> (39.4719, -58.4883) centre (42.3696, -57.7118) ccw
  arc A12 (30.0646, -83.2674) -> (39.7028, -77.7028) centre (24.5, -62.5) ccw
  arc A13 (28.5117, -77.4719) -> (30.0646, -83.2674) centre (29.2882, -80.3696) ccw
  arc A14 (28.5117, -77.4719) -> (35.4602, -73.4602) centre (24.5, -62.5) ccw
  arc A15 (39.7028, -77.7028) -> (35.4602, -73.4602) centre (37.5815, -75.5815) ccw
  arc A16 (34.5896, -34.7791) -> (14.4104, -34.7791) centre (24.5, -62.5) ccw
  arc A17 (32.5375, -40.4172) -> (34.5896, -34.7791) centre (33.5635, -37.5981) ccw
  arc A18 (32.5375, -40.4172) -> (16.4625, -40.4172) centre (24.5, -62.5) ccw
  arc A19 (14.4104, -34.7791) -> (16.4625, -40.4172) centre (15.4365, -37.5981) ccw
  arc A20 (43.4622, -85.0983) -> (53.5518, -67.6226) centre (24.5, -62.5) ccw
  arc A21 (39.6055, -80.502) -> (43.4622, -85.0983) centre (41.5339, -82.8002) ccw
  arc A22 (39.6055, -80.502) -> (47.643, -66.5807) centre (24.5, -62.5) ccw
  arc A23 (53.5518, -67.6226) -> (47.643, -66.5807) centre (50.5974, -67.1017) ccw
  arc A24 (-4.5518, -67.6226) -> (5.5378, -85.0983) centre (24.5, -62.5) ccw
  arc A25 (1.357, -66.5807) -> (-4.5518, -67.6226) centre (-1.5974, -67.1017) ccw
  arc A26 (1.357, -66.5807) -> (9.3945, -80.502) centre (24.5, -62.5) ccw
  arc A27 (5.5378, -85.0983) -> (9.3945, -80.502) centre (7.4661, -82.8002) ccw
  arc A28 (3.7326, -56.9354) -> (3.7326, -68.0646) centre (24.5, -62.5) ccw
  arc A29 (9.5281, -58.4883) -> (3.7326, -56.9354) centre (6.6304, -57.7118) ccw
  arc A30 (9.5281, -58.4883) -> (9.5281, -66.5117) centre (24.5, -62.5) ccw
  arc A31 (3.7326, -68.0646) -> (9.5281, -66.5117) centre (6.6304, -67.2882) ccw
  arc A32 (39.7028, -47.2972) -> (30.0646, -41.7326) centre (24.5, -62.5) ccw
  arc A33 (35.4602, -51.5398) -> (39.7028, -47.2972) centre (37.5815, -49.4185) ccw
  arc A34 (35.4602, -51.5398) -> (28.5117, -47.5281) centre (24.5, -62.5) ccw
  arc A35 (30.0646, -41.7326) -> (28.5117, -47.5281) centre (29.2882, -44.6304) ccw
  arc A36 (9.2972, -77.7028) -> (18.9354, -83.2674) centre (24.5, -62.5) ccw
  arc A37 (13.5398, -73.4602) -> (9.2972, -77.7028) centre (11.4185, -75.5815) ccw
  arc A38 (13.5398, -73.4602) -> (20.4883, -77.4719) centre (24.5, -62.5) ccw
  arc A39 (18.9354, -83.2674) -> (20.4883, -77.4719) centre (19.7118, -80.3696) ccw
  arc A40 (5.5378, -39.9017) -> (-4.5518, -57.3774) centre (24.5, -62.5) ccw
  arc A41 (9.3945, -44.498) -> (5.5378, -39.9017) centre (7.4661, -42.1998) ccw
  arc A42 (9.3945, -44.498) -> (1.357, -58.4193) centre (24.5, -62.5) ccw
  arc A43 (-4.5518, -57.3774) -> (1.357, -58.4193) centre (-1.5974, -57.8983) ccw
  arc A44 (53.5518, -57.3774) -> (43.4622, -39.9017) centre (24.5, -62.5) ccw
  arc A45 (47.643, -58.4193) -> (53.5518, -57.3774) centre (50.5974, -57.8983) ccw
  arc A46 (47.643, -58.4193) -> (39.6055, -44.498) centre (24.5, -62.5) ccw
  arc A47 (43.4622, -39.9017) -> (39.6055, -44.498) centre (41.5339, -42.1998) ccw
  line L0 (-60, 96.1) -> (-60, 112.5)
  line L1 (-60, 112.5) -> (-62, 112.5)
  line L2 (-62, 112.5) -> (-62, -112.5)
  line L3 (-62, -112.5) -> (62, -112.5)
  line L4 (62, -112.5) -> (62, 112.5)
  line L5 (62, 112.5) -> (60, 112.5)
  line L6 (60, 112.5) -> (60, 96.1)
  line L7 (60, 96.1) -> (-60, 96.1)
  circle A48 centre (24.5, -62.5) radius 30
  line L8 (20, -67) -> (29, -67) construction
  line L9 (29, -67) -> (29, -58) construction
  line L10 (29, -58) -> (20, -58) construction
  line L11 (20, -58) -> (20, -67) construction
  line L12 (20, -67) -> (29, -58) construction
  line L13 (29, -67) -> (20, -58) construction
  circle A49 centre (29, -67) radius 2
  circle A50 centre (20, -67) radius 2
  circle A51 centre (20, -58) radius 2
  circle A52 centre (29, -58) radius 2
  point P0 (24.5, -62.5)
  point P1 (24.5, -62.5)
  dimension "d67" = 9
  dimension "d68" = 4
  constraint horizontal L8
  constraint perpendicular L8 L9
  constraint parallel L8 L10
  constraint parallel L9 L11
  constraint coincident L12 P1
  constraint coincident L13 P1
  constraint coincident P1 P0
  constraint equal L8 L11
  constraint coincident L8.end L9.start
  constraint coincident L8.start L11.end
  constraint coincident L10.end L11.start
  constraint coincident L9.end L10.start
  constraint equal A49 A52
  constraint equal A49 A50
  constraint equal A50 A51
  measures "d67" distance of L8.start L8.end
  measures "d68" diameter of A51
extrude "Extrude11" cut sketch "Sketch10" against normal blind 2 contours A49 | A50 | A51 | A52 bodies 1
sketch "Sketch11" plane through (0, 0, 41) normal (0, 0, 1) x (-1, 0, 0)
  circle A0 centre (29, -58) radius 2
  circle A1 centre (29, -67) radius 2
  circle A2 centre (20, -58) radius 2
  circle A3 centre (20, -67) radius 2
  arc A4 (14.4104, -90.2209) -> (34.5896, -90.2209) centre (24.5, -62.5) ccw
  arc A5 (16.4625, -84.5828) -> (14.4104, -90.2209) centre (15.4365, -87.4019) ccw
  arc A6 (16.4625, -84.5828) -> (32.5375, -84.5828) centre (24.5, -62.5) ccw
  arc A7 (34.5896, -90.2209) -> (32.5375, -84.5828) centre (33.5635, -87.4019) ccw
  arc A8 (18.9354, -41.7326) -> (9.2972, -47.2972) centre (24.5, -62.5) ccw
  arc A9 (20.4883, -47.5281) -> (18.9354, -41.7326) centre (19.7118, -44.6304) ccw
  arc A10 (20.4883, -47.5281) -> (13.5398, -51.5398) centre (24.5, -62.5) ccw
  arc A11 (9.2972, -47.2972) -> (13.5398, -51.5398) centre (11.4185, -49.4185) ccw
  arc A12 (45.2674, -68.0646) -> (45.2674, -56.9354) centre (24.5, -62.5) ccw
  arc A13 (39.4719, -66.5117) -> (45.2674, -68.0646) centre (42.3696, -67.2882) ccw
  arc A14 (39.4719, -66.5117) -> (39.4719, -58.4883) centre (24.5, -62.5) ccw
  arc A15 (45.2674, -56.9354) -> (39.4719, -58.4883) centre (42.3696, -57.7118) ccw
  arc A16 (30.0646, -83.2674) -> (39.7028, -77.7028) centre (24.5, -62.5) ccw
  arc A17 (28.5117, -77.4719) -> (30.0646, -83.2674) centre (29.2882, -80.3696) ccw
  arc A18 (28.5117, -77.4719) -> (35.4602, -73.4602) centre (24.5, -62.5) ccw
  arc A19 (39.7028, -77.7028) -> (35.4602, -73.4602) centre (37.5815, -75.5815) ccw
  arc A20 (34.5896, -34.7791) -> (14.4104, -34.7791) centre (24.5, -62.5) ccw
  arc A21 (32.5375, -40.4172) -> (34.5896, -34.7791) centre (33.5635, -37.5981) ccw
  arc A22 (32.5375, -40.4172) -> (16.4625, -40.4172) centre (24.5, -62.5) ccw
  arc A23 (14.4104, -34.7791) -> (16.4625, -40.4172) centre (15.4365, -37.5981) ccw
  arc A24 (43.4622, -85.0983) -> (53.5518, -67.6226) centre (24.5, -62.5) ccw
  arc A25 (39.6055, -80.502) -> (43.4622, -85.0983) centre (41.5339, -82.8002) ccw
  arc A26 (39.6055, -80.502) -> (47.643, -66.5807) centre (24.5, -62.5) ccw
  arc A27 (53.5518, -67.6226) -> (47.643, -66.5807) centre (50.5974, -67.1017) ccw
  arc A28 (-4.5518, -67.6226) -> (5.5378, -85.0983) centre (24.5, -62.5) ccw
  arc A29 (1.357, -66.5807) -> (-4.5518, -67.6226) centre (-1.5974, -67.1017) ccw
  arc A30 (1.357, -66.5807) -> (9.3945, -80.502) centre (24.5, -62.5) ccw
  arc A31 (5.5378, -85.0983) -> (9.3945, -80.502) centre (7.4661, -82.8002) ccw
  arc A32 (3.7326, -56.9354) -> (3.7326, -68.0646) centre (24.5, -62.5) ccw
  arc A33 (9.5281, -58.4883) -> (3.7326, -56.9354) centre (6.6304, -57.7118) ccw
  arc A34 (9.5281, -58.4883) -> (9.5281, -66.5117) centre (24.5, -62.5) ccw
  arc A35 (3.7326, -68.0646) -> (9.5281, -66.5117) centre (6.6304, -67.2882) ccw
  arc A36 (39.7028, -47.2972) -> (30.0646, -41.7326) centre (24.5, -62.5) ccw
  arc A37 (35.4602, -51.5398) -> (39.7028, -47.2972) centre (37.5815, -49.4185) ccw
  arc A38 (35.4602, -51.5398) -> (28.5117, -47.5281) centre (24.5, -62.5) ccw
  arc A39 (30.0646, -41.7326) -> (28.5117, -47.5281) centre (29.2882, -44.6304) ccw
  arc A40 (9.2972, -77.7028) -> (18.9354, -83.2674) centre (24.5, -62.5) ccw
  arc A41 (13.5398, -73.4602) -> (9.2972, -77.7028) centre (11.4185, -75.5815) ccw
  arc A42 (13.5398, -73.4602) -> (20.4883, -77.4719) centre (24.5, -62.5) ccw
  arc A43 (18.9354, -83.2674) -> (20.4883, -77.4719) centre (19.7118, -80.3696) ccw
  arc A44 (5.5378, -39.9017) -> (-4.5518, -57.3774) centre (24.5, -62.5) ccw
  arc A45 (9.3945, -44.498) -> (5.5378, -39.9017) centre (7.4661, -42.1998) ccw
  arc A46 (9.3945, -44.498) -> (1.357, -58.4193) centre (24.5, -62.5) ccw
  arc A47 (-4.5518, -57.3774) -> (1.357, -58.4193) centre (-1.5974, -57.8983) ccw
  arc A48 (53.5518, -57.3774) -> (43.4622, -39.9017) centre (24.5, -62.5) ccw
  arc A49 (47.643, -58.4193) -> (53.5518, -57.3774) centre (50.5974, -57.8983) ccw
  arc A50 (47.643, -58.4193) -> (39.6055, -44.498) centre (24.5, -62.5) ccw
  arc A51 (43.4622, -39.9017) -> (39.6055, -44.498) centre (41.5339, -42.1998) ccw
  line L0 (-60, 96.1) -> (-60, 112.5)
  line L1 (-60, 112.5) -> (-62, 112.5)
  line L2 (-62, 112.5) -> (-62, -112.5)
  line L3 (-62, -112.5) -> (62, -112.5)
  line L4 (62, -112.5) -> (62, 112.5)
  line L5 (62, 112.5) -> (60, 112.5)
  line L6 (60, 112.5) -> (60, 96.1)
  line L7 (60, 96.1) -> (-60, 96.1)
  line L8 (62, 41.8) -> (-62, 41.8) construction
  line L9 (42.3, 41.8) -> (42.3, 39.3) construction
  line L10 (12.3, 41.8) -> (12.3, 39.3) construction
  line L11 (42.3, 41.8) -> (42.3, 44.3) construction
  line L12 (12.3, 41.8) -> (12.3, 44.3) construction
  line L13 (42.3, 39.3) -> (12.3, 39.3)
  line L14 (12.3, 44.3) -> (42.3, 44.3)
  arc A52 (42.3, 39.3) -> (42.3, 44.3) centre (42.3, 41.8) ccw
  arc A53 (12.3, 44.3) -> (12.3, 39.3) centre (12.3, 41.8) ccw
  line L15 (42.3, 41.8) -> (42.3, 15.1224) construction
  line L16 (42.3, 41.8) -> (42.3, 79.2423) construction
  line L17 (42.3, 29.3) -> (12.3, 29.3)
  arc A54 (42.3, 29.3) -> (42.3, 34.3) centre (42.3, 31.8) ccw
  line L18 (12.3, 34.3) -> (42.3, 34.3)
  arc A55 (12.3, 34.3) -> (12.3, 29.3) centre (12.3, 31.8) ccw
  line L19 (42.3, 19.3) -> (12.3, 19.3)
  arc A56 (42.3, 19.3) -> (42.3, 24.3) centre (42.3, 21.8) ccw
  line L20 (12.3, 24.3) -> (42.3, 24.3)
  arc A57 (12.3, 24.3) -> (12.3, 19.3) centre (12.3, 21.8) ccw
  line L21 (12.3, 74.3) -> (42.3, 74.3)
  arc A58 (42.3, 69.3) -> (42.3, 74.3) centre (42.3, 71.8) ccw
  line L22 (42.3, 69.3) -> (12.3, 69.3)
  arc A59 (12.3, 74.3) -> (12.3, 69.3) centre (12.3, 71.8) ccw
  arc A60 (-45.7, 34.3) -> (-45.7, 29.3) centre (-45.7, 31.8) ccw
  line L23 (-45.7, 34.3) -> (-15.7, 34.3)
  arc A61 (-15.7, 29.3) -> (-15.7, 34.3) centre (-15.7, 31.8) ccw
  line L24 (-15.7, 29.3) -> (-45.7, 29.3)
  dimension "d71" = 5
  dimension "d72" = 30
  dimension "d73" = 19.7
  dimension "d76" = 0
  dimension "d77" = -10
  dimension "d80" = 0
  dimension "d81" = 30
  dimension "d82" = 21.8
  dimension "d85" = -58
  dimension "d86" = 0
  constraint coincident L4 L8.start
  constraint coincident L2 L8.end
  constraint perpendicular L2 L8
  constraint coincident L8 L9.start
  constraint coincident L8 L10.start
  constraint equal A52 A53
  constraint coincident L9.start L11.start
  constraint perpendicular L8 L9
  constraint coincident L10.start L12.start
  constraint perpendicular L8 L10
  constraint parallel L10 L11
  constraint perpendicular L8 L12
  constraint tangent L14 A53
  constraint perpendicular L13 L15
  constraint perpendicular L14 L16
  measures "d71" diameter of A53
  measures "d72" distance of L9.start L10.start
  measures "d73" distance of L4 L9.start
  measures "d82" distance of L7 L21
extrude "Extrude12" cut sketch "Sketch11" against normal blind 2 contours L13 L14 A52 A53 | L17 A54 L18 A55 | L19 A56 L20 A57 | L21 A58 L22 A59 | A60 L23 A61 L24 bodies 1